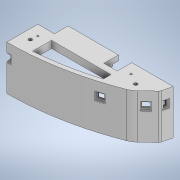
# Autodesk Inventor part: bumper_base_final _원본수정
Saved by Autodesk Inventor 2020 (Build 240168000, 168)
## iProperties
Created: 2022-06-30
Part Number: bumper_base_final _원본수정
Material: 일반
Document SubType Name: Modeling
Designer: samsung
Density: 1 g/cm^3
Appearance: 기본값
Author: samsung
Autodesk Inventor part; units mm, degrees
sketch "스케치1" plane through (0, 0, 0) normal (0, 1, 0) x (-1, 0, 0)
  line L0 (-417.5, 136.0278) -> (167.5, 136.0278)
  line L1 (143.8982, 68.5278) -> (-85, 68.5278)
  line L2 (-165, 68.5278) -> (-381.3624, 68.5278)
  line L3 (-125, -531.4722) -> (-125, 1435.9267)
  circle A0 centre (-125, -531.4722) radius 1967.3989
  line L4 (-125, 111.6599) -> (186.953, 1411.0375)
  line L5 (-417.5444, 28.5399) -> (-411.5443, 53.4914)
  arc A1 (1441.9544, 38.2515) -> (-1691.7763, 38.7413) centre (-125, -531.4722) ccw
  line L6 (-371.3038, 78.1512) -> (-261.7019, 111.6599)
  line L7 (-261.7019, 111.6599) -> (11.7019, 111.6599)
  line L8 (-316.5029, 94.9056) -> (-320.1581, 106.8613)
  line L9 (-407.5098, 28.5399) -> (-405.1717, 38.2627)
  line L10 (-405.1717, 38.2627) -> (-402.8337, 47.9856)
  line L11 (-402.8337, 47.9856) -> (-371.3038, 78.1512)
  line L12 (-125, -531.4722) -> (-261.7019, 111.6599)
  line L13 (-125, -531.4722) -> (11.7019, 111.6599)
  line L14 (-417.5444, 28.5399) -> (-407.5098, 28.5399)
  line L15 (-125, -531.4722) -> (-371.3038, 78.1512)
  line L16 (-125, -531.4722) -> (121.3038, 78.1512)
  line L17 (11.7019, 111.6599) -> (121.3038, 78.1512)
  line L18 (167.4556, 28.5399) -> (156.6099, 73.7155)
  line L19 (157.5156, 28.5399) -> (148.4052, 66.4876)
  line L20 (121.3038, 78.1512) -> (152.8486, 47.9794)
  line L21 (155.1841, 38.2515) -> (1758.102, 38.2515)
  line L22 (155.1841, 38.2515) -> (164.5823, 40.5079)
  line L23 (157.5156, 28.5399) -> (167.4556, 28.5399)
  line L24 (155.1841, 38.2515) -> (1422.1711, 683.8137)
  line L25 (66.5029, 94.9056) -> (70.1581, 106.8613)
  line L26 (66.5029, 94.9056) -> (738.7616, 1236.1743)
  line L27 (66.5029, 94.9056) -> (147.3646, 1416.9826)
  line L28 (137.0762, 63.0653) -> (150.1137, 76.6961)
  line L29 (137.0762, 63.0653) -> (801.7772, 1203.965)
  line L30 (137.0762, 63.0653) -> (1307.7755, 816.7906)
  line L31 (-125, -531.4722) -> (148.4052, 66.4876)
  line L32 (-259.0118, 93.6599) -> (9.0118, 93.6599)
  line L33 (111.9521, 62.1879) -> (136.5817, 38.6304)
  line L34 (9.0118, 93.6599) -> (111.9521, 62.1879)
  line L35 (-361.9509, 62.1883) -> (-386.641, 38.5664)
  line L36 (-387.0049, 38.256) -> (-387.0101, 38.2515)
  line L37 (-388.9967, 28.5399) -> (-386.569, 38.6353)
  line L38 (-361.9509, 62.1883) -> (-259.0118, 93.6599)
  line L39 (-407.5098, 28.5399) -> (-388.9967, 28.5399)
  line L40 (136.5817, 38.6304) -> (139.0042, 28.5399)
  line L41 (157.5156, 28.5399) -> (139.0042, 28.5399)
  line L42 (-125, 111.6599) -> (-155, 111.6599)
  line L43 (-155, 93.6599) -> (-125, 93.6599)
  line L44 (-125, 93.6599) -> (-125, 111.6599)
  line L45 (-376.8352, 86.6988) -> (-411.5443, 53.4914)
  arc A2 (156.6099, 73.7155) -> (-376.8352, 86.6988) centre (-125, -531.4722) ccw
  arc A3 (148.4052, 66.4876) -> (-371.3038, 78.1512) centre (-125, -531.4722) ccw
  arc A4 (-398.3819, 66.4982) -> (-398.3844, 66.4971) centre (-125, -531.4722) ccw
  line L46 (-407.5098, 28.5399) -> (-402.8337, 47.9856)
  line L47 (-398.3829, 66.4939) -> (-398.3801, 66.5058)
  line L48 (-398.3844, 66.4971) -> (-398.2523, 66.2083)
  line L49 (-393.8505, 56.5801) -> (-125, -531.4722)
  line L50 (-125, 111.6599) -> (-135, 111.6599)
  line L51 (-135, 111.6599) -> (-135, 103.6599)
  line L52 (-135, 103.6599) -> (-125, 103.6599)
  line L53 (-316.5029, 94.9056) -> (-326.0659, 91.9818)
  line L54 (-326.0659, 91.9818) -> (-323.727, 84.3314)
  line L55 (-323.727, 84.3314) -> (-304.6009, 90.1788)
  line L56 (-304.6009, 90.1788) -> (-306.9398, 97.8293)
  line L57 (-402.8337, 47.9856) -> (-395.0554, 46.1151)
  line L58 (-395.0554, 46.1151) -> (-398.5625, 31.5309)
  line L59 (-398.5625, 31.5309) -> (-406.3408, 33.4013)
  line L60 (-387.0687, 63.0684) -> (-394.2944, 56.1554)
  line L61 (-394.2944, 56.1554) -> (-388.764, 50.3749)
  line L62 (-388.764, 50.3749) -> (-374.3127, 64.2009)
  line L63 (-374.3127, 64.2009) -> (-379.8431, 69.9814)
  line L64 (-165, 0) -> (-165, 124.81)
  line L65 (-341.215, 68.5278) -> (-341.215, 89.4604)
  line L66 (-388.9967, 28.5399) -> (-125, 28.5399)
  line L67 (-125, 0) -> (-165, 0)
  line L68 (-175, 28.5399) -> (-175, 124.1239)
  line L69 (-165, 0) -> (-135, 0)
  line L70 (-135, 0) -> (-135, 61.5)
  line L71 (-135, 61.5) -> (-165, 61.5)
  line L72 (-165, 61.5) -> (-165, 0)
  line L73 (-165, 61.5) -> (-175, 61.5)
  line L74 (-135, 61.5) -> (-125, 61.5)
  line L75 (-175, 78.5399) -> (-370.0325, 78.5399)
  line L76 (-318, 28.5399) -> (-318, 97.0636)
  line L77 (-286, 28.5399) -> (-286, 89.4604)
  line L78 (-318, 28.5399) -> (-318, 94.4478)
  line L79 (-286, 28.5399) -> (-318, 28.5399)
  line L80 (-318, 28.5399) -> (-318, 63.5399)
  line L81 (-318, 63.5399) -> (-286, 63.5399)
  line L82 (-286, 63.5399) -> (-286, 28.5399)
  point P0 (0, 0)
  point P1 (0, 0)
  point P2 (143.8982, 61.5)
  point P3 (-393.8982, 61.5)
  point P4 (-417.5, 21.5)
  point P5 (-165, 0)
  point P6 (-85, 0)
  point P7 (-85, 12.4229)
  point P8 (167.5, 12.4229)
  point P9 (-393.8982, -388.5)
  point P10 (-165, -388.5)
  point P11 (167.5, -327)
  point P12 (-417.5, -327)
  point P13 (-85, -388.5)
  point P14 (143.8982, -388.5)
  point P15 (162, 21.5)
  point P16 (162, 12.4229)
  point P17 (167.5, 21.5)
  point P18 (-125, 0)
  point P19 (-125, 136.0278)
  point P20 (-125, 136.0278)
  point P21 (-125, 93.6599)
  point P22 (-125, 126.0278)
  point P23 (-317.2344, 97.2982)
  point P24 (-378.4524, 68.5278)
  point P25 (-393.0723, 54.878)
  point P26 (-175, 68.5278)
  point P27 (-341.215, 78.5399)
  point P28 (-351.2596, 28.5399)
  point P29 (-318, 68.5278)
  point P30 (-318, 94.4478)
  point P31 (-165, 28.5399)
  point P32 (-308.467, 78.5399)
  point P33 (-318, 75.6254)
  point P34 (-318, 78.5399)
  point P35 (-286, 68.5278)
  dimension "d15" = 585
  dimension "d31" = 13.5
  dimension "d56" = 12
  dimension "d57" = 12
  dimension "d60" = 10
  dimension "d65" = 13.5
  dimension "d66" = 13.5
  dimension "d68" = 13.5
  dimension "d69" = 13.5
  dimension "d70" = 13.5
  dimension "d71" = 13.5
  dimension "d72" = 10
  dimension "d81" = 18
  dimension "d83" = 18
  dimension "d84" = 18
  dimension "d85" = 18
  dimension "d86" = 18
  dimension "d159" = 10
  dimension "d164" = 10
  dimension "d165" = 8
  dimension "d166" = 10
  dimension "d167" = 8
  dimension "d168" = 20
  dimension "d169" = 8
  dimension "d170" = 15
  dimension "d171" = 10
  dimension "d172" = 8
  dimension "d173" = 20
  dimension "d191" = 30
  dimension "d192" = 61.5
  dimension "d194" = 50
  dimension "d256" = 143
  dimension "d264" = 121
  dimension "d265" = 32
  dimension "d266" = 35
  constraints: 166 end point, 33 point on line, 22 perpendicular, 14 parallel, 11 horizontal, 10 point on circle, 7 midpoint, 3 centre point, 2 vertical, 1 coincident, 1 tangent, 23 other
  measures "d15" distance of L18.start L5.start
  measures "d31" angle of L4 L3
  measures "d56" angle of L3 L12
  measures "d57" angle of L13 L3
  measures "d60" angle of L15 L12
  measures "d65" angle of L22 L21
  measures "d66" angle of L24 L22
  measures "d68" angle of L26 L25
  measures "d69" angle of L25 L27
  measures "d70" angle of L29 L28
  measures "d71" angle of L30 L28
  measures "d72" angle of L16 L13
  measures "d81" distance between parallel lines of L7 L32
  measures "d83" distance between parallel lines of L20 L33
  measures "d84" distance between parallel lines of L11 L35
  measures "d85" distance between parallel lines of L9 L37
  measures "d86" distance between parallel lines of L19 L40
  measures "d159" distance between parallel lines of L11 L45
  measures "d164" distance of L4.start L50.end
  measures "d165" distance of L50.end L51.end
  measures "d166" distance of L8.start L53.end
  measures "d167" distance of L53.end L54.end
  measures "d168" distance of L54.end L55.end
  measures "d169" distance of L10.end L57.end
  measures "d170" distance of L57.end L58.end
  measures "d171" distance of L60.start L60.end
  measures "d172" distance of L60.end L61.end
  measures "d173" distance of L61.end L62.end
  measures "d191" distance of L71.end L70.end
  measures "d192" distance of L70.end L69.end
  measures "d194" distance between parallel lines of L66 L75
  measures "d256" distance between parallel lines of L68 L76
  measures "d264" distance between parallel lines of L77 L64
  measures "d265" distance between parallel lines of L78 L77
  measures "d266" distance of L79.end L80.end
extrude "돌출11" add sketch "스케치1" against normal blind 90 contours L3 A3 L8 A2 | L8 A3 L11 L10 L9 L14 L5 L45 A2
ref_plane "작업 평면1" through (125, 0, 103.6599) normal (0, 0, 1) x (1, 0, 0)
sketch "스케치14" plane through (125, 0, 103.6599) normal (0, 0, 1) x (1, 0, 0)
  line L0 (0, 0) -> (10, 0) projected
  line L1 (10, -30) -> (0, -30) projected
  line L2 (7.5, -7.5) -> (-7.5, -7.5)
  line L3 (-7.5, -7.5) -> (-7.5, -22.5)
  line L4 (-7.5, -22.5) -> (7.5, -22.5)
  line L5 (7.5, -22.5) -> (7.5, -7.5)
  line L6 (7.5, -7.5) -> (-7.5, -22.5) construction
  line L7 (-7.5, -7.5) -> (7.5, -22.5) construction
  line L8 (0, -7.5) -> (0, -22.5)
  point P0 (0, -15)
  dimension "d236" = 15
  dimension "d237" = 15
  constraints: 14 end point, 4 midpoint, 2 parallel, 1 horizontal, 1 perpendicular
  measures "d236" distance of L4.end L3.end
  measures "d237" distance of L3.end L2.end
extrude "돌출13" cut sketch "스케치14" along normal blind 50 contours L5 L4 L8 L2
ref_plane "작업 평면2" through (304.6009, -30, 90.1788) normal (0.2923717, 0, 0.9563048) x (0.9563048, 0, -0.2923717)
sketch "스케치15" plane through (304.6009, -30, 90.1788) normal (0.2923717, 0, 0.9563048) x (0.9563048, 0, -0.2923717)
  line L0 (0, 30) -> (20, 30)
  line L1 (0, 30) -> (0, 0)
  line L2 (20, 0) -> (0, 0)
  line L3 (20, 30) -> (20, 0)
  line L4 (2.5, 22.5) -> (17.5, 22.5)
  line L5 (17.5, 22.5) -> (17.5, 7.5)
  line L6 (17.5, 7.5) -> (2.5, 7.5)
  line L7 (2.5, 7.5) -> (2.5, 22.5)
  line L8 (2.5, 22.5) -> (17.5, 7.5) construction
  line L9 (17.5, 22.5) -> (2.5, 7.5) construction
  point P0 (-264.9255, 30)
  point P1 (10, 15)
  dimension "d234" = 15
  dimension "d235" = 15
  constraints: 20 end point, 2 midpoint, 2 parallel, 1 horizontal, 1 perpendicular
  measures "d234" distance of L5.end L6.end
  measures "d235" distance of L4.end L5.end
extrude "돌출14" cut sketch "스케치15" along normal blind 50 contours L4 L5 L6 L7
ref_plane "작업 평면3" through (374.3127, -30, 64.2009) normal (0.6913026, 0, 0.7225653) x (0.7225653, 0, -0.6913026)
sketch "스케치16" plane through (374.3127, -30, 64.2009) normal (0.6913026, 0, 0.7225653) x (0.7225653, 0, -0.6913026)
  line L0 (0, 30) -> (20, 30)
  line L1 (0, 30) -> (0, 0)
  line L2 (20, 0) -> (0, 0)
  line L3 (20, 30) -> (20, 0)
  line L4 (2.5, 22.5) -> (17.5, 22.5)
  line L5 (17.5, 22.5) -> (17.5, 7.5)
  line L6 (17.5, 7.5) -> (2.5, 7.5)
  line L7 (2.5, 7.5) -> (2.5, 22.5)
  line L8 (2.5, 22.5) -> (17.5, 7.5) construction
  line L9 (17.5, 22.5) -> (2.5, 7.5) construction
  point P0 (-226.0831, 30)
  point P1 (10, 15)
  dimension "d232" = 15
  dimension "d233" = 15
  constraints: 20 end point, 2 midpoint, 2 parallel, 1 horizontal, 1 perpendicular
  measures "d232" distance of L5.end L6.end
  measures "d233" distance of L4.end L5.end
extrude "돌출15" cut sketch "스케치16" along normal blind 50 contours L4 L5 L6 L7
ref_plane "작업 평면4" through (395.0554, -30, 46.1151) normal (0.972283, 0, 0.233807) x (0.233807, 0, -0.972283)
sketch "스케치17" plane through (395.0554, -30, 46.1151) normal (0.972283, 0, 0.233807) x (0.233807, 0, -0.972283)
  line L0 (0, 30) -> (15, 30)
  line L1 (0, 30) -> (0, 0)
  line L2 (15, 0) -> (0, 0)
  line L3 (15, 30) -> (15, 0)
  line L4 (11.5, 22.5) -> (3.5, 22.5)
  line L5 (3.5, 22.5) -> (3.5, 7.5)
  line L6 (3.5, 7.5) -> (11.5, 7.5)
  line L7 (11.5, 7.5) -> (11.5, 22.5)
  line L8 (11.5, 22.5) -> (3.5, 7.5) construction
  line L9 (3.5, 22.5) -> (11.5, 7.5) construction
  point P0 (7.5, 15)
  point P1 (7.5, 15)
  point P2 (15, 15)
  dimension "d230" = 8
  dimension "d231" = 15
  constraints: 20 end point, 4 midpoint, 2 parallel, 1 horizontal, 1 horizontal alignment, 1 perpendicular, 4 other
  measures "d230" distance of L6.end L5.end
  measures "d231" distance of L5.end L4.end
extrude "돌출16" cut sketch "스케치17" along normal blind 50 contours L7 L6 L5 L4
extrude "돌출17" add sketch "스케치1" along normal blind 17 contours L3 A3 L8 A2 | L3 L7 L64 A3 | L8 A3 L11 L10 L9 L14 L5 L45 A2 | L3 L52 L51 L7 | L64 L7 L68 A3 | L3 L32 L64 L7 L51 L52 | L64 L32 L68 L7 | L76 L6 L65 A3 | L3 L74 L71 L64 L32 | L64 L2 L68 L32 | L76 L55 L54 L6 | L65 L6 A3 | L64 L73 L68 L2 | L54 L55 L76 L75 L65 L6 | L75 L68 L2 L12 | L12 L2 L77 L75 | L15 L2 L63 L11 | L6 L75 L65 L2 L15 | L65 L75 L6 | L68 L66 L12 L2 | L64 L66 L68 L73 | L76 L38 L65 L75 | L75 L38 L76 | L12 L66 L77 L2 | L77 L2 L76 L38 L75 | L63 L2 L11 | L15 L35 L49 L61 L62 L63 L2 | L2 L38 L35 L15 | L9 L59 L58 L57 L11 L61 L49 L35 L37 L39 | L66 L49 L35 L15 | L15 L35 L38 L2 L76 L66 | L66 L37 L35 L49 | L76 L2 L38 | L77 L81 L76 L2 | L2 L63 L62 L61 L49 L11 | L9 L10 L57 L58 L59 | L61 L11 L49
sketch "스케치18" plane through (0, 17, 0) normal (0, 1, 0) x (1, 0, 0)
  line L0 (407.5098, -28.5399) -> (402.8337, -47.9856) projected
  line L1 (402.8337, -47.9856) -> (371.3038, -78.1512) projected
  arc A0 (125, -126.0278) -> (371.3038, -78.1512) centre (125, 531.4722) ccw projected
  line L2 (417.5444, -28.5399) -> (318, -28.5399) projected
  circle A1 centre (367.5098, -68.5399) radius 3.6
  line L3 (369.5883, -64.9399) -> (371.6667, -68.5399)
  line L4 (371.6667, -68.5399) -> (369.5883, -72.1399)
  line L5 (369.5883, -72.1399) -> (365.4313, -72.1399)
  line L6 (365.4313, -72.1399) -> (363.3529, -68.5399)
  line L7 (363.3529, -68.5399) -> (365.4313, -64.9399)
  line L8 (365.4313, -64.9399) -> (369.5883, -64.9399)
  line L9 (261.7019, -111.6599) -> (-11.7019, -111.6599) projected
  line L10 (259.0118, -93.6599) -> (-9.0118, -93.6599) projected
  line L11 (125, 531.4722) -> (125, -126.0278) projected
  line L12 (125, 202.7222) -> (125, -111.6599)
  circle A2 centre (148, -102.6599) radius 3.6
  line L13 (150.0785, -99.0599) -> (152.1569, -102.6599)
  line L14 (152.1569, -102.6599) -> (150.0785, -106.2599)
  line L15 (150.0785, -106.2599) -> (145.9215, -106.2599)
  line L16 (145.9215, -106.2599) -> (143.8431, -102.6599)
  line L17 (143.8431, -102.6599) -> (145.9215, -99.0599)
  line L18 (145.9215, -99.0599) -> (150.0785, -99.0599)
  point P0 (0, 0)
  point P1 (341.215, -89.4604)
  point P2 (165, -28.5399)
  point P3 (367.5098, -64.9399)
  point P4 (125, -61.5)
  point P5 (148, -99.0599)
  point P6 (175, -124.1239)
  point P7 (351.2596, -28.5399)
  dimension "d197" = 7.2
  dimension "d229" = 7.2
  dimension "d195" = 40
  dimension "d196" = 40
  dimension "d224" = 9
  dimension "d225" = 23
  constraints: 26 end point, 5 coincident, 4 midpoint, 2 vertical alignment, 1 point on line, 30 other
  measures "d195" horizontal distance of point (367.51, -68.54) L0.start
  measures "d196" horizontal distance of L0.start point (367.51, -68.54)
  measures "d224" distance from line of point (148, -102.66) L9
  measures "d225" distance from line of point (148, -102.66) L11
extrude "돌출18" cut sketch "스케치18" against normal blind 10 contours A1 | A1 L3 L4 | A1 L8 L3 | L4 L5 A1 | A1 L7 L8 | L5 L6 A1 | A1 L6 L7 | A2 | A2 L13 L14 | A2 L18 L13 | L14 L15 A2 | A2 L17 L18 | L15 L16 A2 | A2 L16 L17
sketch "스케치19" plane through (0, 7, 0) normal (0, 1, 0) x (1, 0, 0)
  line L0 (363.3529, -68.5399) -> (365.4313, -64.9399) projected
  line L1 (365.4313, -72.1399) -> (363.3529, -68.5399) projected
  line L2 (369.5883, -72.1399) -> (365.4313, -72.1399) projected
  line L3 (371.6667, -68.5399) -> (369.5883, -72.1399) projected
  line L4 (369.5883, -64.9399) -> (371.6667, -68.5399) projected
  line L5 (365.4313, -64.9399) -> (369.5883, -64.9399) projected
  line L6 (125, -61.5) -> (125, -126.0278) projected
  line L7 (261.7019, -111.6599) -> (-11.7019, -111.6599) projected
  line L8 (259.0118, -93.6599) -> (-9.0118, -93.6599) projected
  line L9 (152.1569, -102.6599) -> (150.0785, -106.2599) projected
  line L10 (150.0785, -99.0599) -> (152.1569, -102.6599) projected
  line L11 (145.9215, -99.0599) -> (150.0785, -99.0599) projected
  line L12 (143.8431, -102.6599) -> (145.9215, -99.0599) projected
  line L13 (145.9215, -106.2599) -> (143.8431, -102.6599) projected
  line L14 (150.0785, -106.2599) -> (145.9215, -106.2599) projected
  point P0 (0, 0)
  point P1 (367.5098, -68.5399)
  point P2 (148, -102.6599)
  point P3 (125, 531.4722)
  point P4 (125, 0)
  point P5 (125, -28.5399)
  dimension "d227" = 23
  dimension "d228" = 9
  measures "d227" distance from line of L6 point (148, -102.66)
  measures "d228" distance from line of L8 point (148, -102.66)
hole "구멍3" at (367.5098, 7, 68.5399) at (148, 7, 102.6599) direction (0, -1, 0) diameter 4.2 end through all
sketch "스케치20" plane through (0, 0, 0) normal (0, -1, 0) x (1, 0, 0)
  circle A0 centre (367.5098, 68.5399) radius 2.1 projected
  arc A1 (175, 124.1239) -> (125, 126.0278) centre (125, -531.4722) ccw projected
  line L0 (125, 61.5) -> (125, 126.0278) projected
  line L1 (407.5098, 28.5399) -> (402.8337, 47.9856) projected
  line L2 (402.8337, 47.9856) -> (371.3038, 78.1512) projected
  circle A2 centre (150, 86.5) radius 3.6
  circle A3 centre (341.215, 53.5399) radius 3.6
  line L3 (152.0785, 90.1) -> (154.1569, 86.5)
  line L4 (154.1569, 86.5) -> (152.0785, 82.9)
  line L5 (152.0785, 82.9) -> (147.9215, 82.9)
  line L6 (147.9215, 82.9) -> (145.8431, 86.5)
  line L7 (145.8431, 86.5) -> (147.9215, 90.1)
  line L8 (147.9215, 90.1) -> (152.0785, 90.1)
  line L9 (343.2935, 57.1399) -> (345.372, 53.5399)
  line L10 (345.372, 53.5399) -> (343.2935, 49.9399)
  line L11 (343.2935, 49.9399) -> (339.1366, 49.9399)
  line L12 (339.1366, 49.9399) -> (337.0581, 53.5399)
  line L13 (337.0581, 53.5399) -> (339.1366, 57.1399)
  line L14 (339.1366, 57.1399) -> (343.2935, 57.1399)
  line L15 (175, 124.1239) -> (175, 78.5399) projected
  arc A4 (371.3038, 78.1512) -> (318, 97.0636) centre (125, -531.4722) ccw projected
  line L16 (165, 61.5) -> (125, 61.5) projected
  circle A5 centre (148, 102.6599) radius 2.1 projected
  line L17 (165, 28.5399) -> (165, 61.5) projected
  line L18 (286, 28.5399) -> (165, 28.5399) projected
  line L19 (175, 78.5399) -> (318, 78.5399) projected
  line L20 (286, 63.5399) -> (286, 28.5399) projected
  line L21 (407.5098, 28.5399) -> (318, 28.5399) projected
  line L22 (318, 63.5399) -> (286, 63.5399) projected
  line L23 (318, 28.5399) -> (318, 63.5399) projected
  line L24 (318, 78.5399) -> (318, 97.0636) projected
  point P0 (0, 0)
  point P1 (341.215, 84.0002)
  point P2 (150, 90.1)
  point P3 (341.215, 57.1399)
  dimension "d212" = 7.2
  dimension "d213" = 7.2
  dimension "d259" = 25
  dimension "d263" = 25
  constraints: 24 end point, 5 coincident, 3 vertical alignment, 2 midpoint, 30 other
  measures "d259" distance from line of L0 point (150, 86.5)
  measures "d263" distance from line of L16 point (150, 86.5)
extrude "돌출19" cut sketch "스케치20" against normal blind 10 contours A2 | A2 L3 L4 | A2 L8 L3 | L4 L5 A2 | A2 L7 L8 | L5 L6 A2 | A2 L6 L7 | A3 | A3 L9 L10 | A3 L14 L9 | L10 L11 A3 | A3 L13 L14 | L11 L12 A3 | A3 L12 L13
sketch "스케치21" plane through (0, 10, 0) normal (0, -1, 0) x (1, 0, 0)
  line L0 (147.9215, 90.1) -> (152.0785, 90.1) projected
  line L1 (145.8431, 86.5) -> (147.9215, 90.1) projected
  line L2 (147.9215, 82.9) -> (145.8431, 86.5) projected
  line L3 (152.0785, 82.9) -> (147.9215, 82.9) projected
  line L4 (154.1569, 86.5) -> (152.0785, 82.9) projected
  line L5 (152.0785, 90.1) -> (154.1569, 86.5) projected
  line L6 (339.1366, 49.9399) -> (337.0581, 53.5399) projected
  line L7 (343.2935, 49.9399) -> (339.1366, 49.9399) projected
  line L8 (345.372, 53.5399) -> (343.2935, 49.9399) projected
  line L9 (343.2935, 57.1399) -> (345.372, 53.5399) projected
  line L10 (339.1366, 57.1399) -> (343.2935, 57.1399) projected
  line L11 (337.0581, 53.5399) -> (339.1366, 57.1399) projected
  circle A0 centre (148, 102.6599) radius 2.1 projected
  arc A1 (175, 124.1239) -> (125, 126.0278) centre (125, -531.4722) ccw projected
  line L12 (125, 61.5) -> (125, 126.0278) projected
  line L13 (165, 61.5) -> (125, 61.5) projected
  line L14 (175, 124.1239) -> (175, 78.5399) projected
  line L15 (165, 28.5399) -> (165, 61.5) projected
  line L16 (286, 28.5399) -> (165, 28.5399) projected
  line L17 (407.5098, 28.5399) -> (402.8337, 47.9856) projected
  line L18 (402.8337, 47.9856) -> (371.3038, 78.1512) projected
  arc A2 (371.3038, 78.1512) -> (318, 97.0636) centre (125, -531.4722) ccw projected
  line L19 (175, 78.5399) -> (318, 78.5399) projected
  line L20 (286, 63.5399) -> (286, 28.5399) projected
  line L21 (407.5098, 28.5399) -> (318, 28.5399) projected
  line L22 (318, 63.5399) -> (286, 63.5399) projected
  line L23 (318, 28.5399) -> (318, 63.5399) projected
  line L24 (318, 78.5399) -> (318, 97.0636) projected
  point P0 (0, 0)
  point P1 (150, 86.5)
  point P2 (341.215, 53.5399)
  dimension "d260" = 25
  dimension "d261" = 25
  measures "d260" distance from line of L12 point (150, 86.5)
  measures "d261" distance from line of L13 point (150, 86.5)
hole "구멍4" at (150, 10, 86.5) at (341.215, 10, 53.5399) direction (0, 1, 0) diameter 4.2 end through all
sketch "스케치22" plane through (411.5443, -90, 53.4914) normal (0.972283, 0, 0.233807) x (0.233807, 0, -0.972283)
  line L0 (6.8166, 82.5) -> (14.8166, 82.5) projected
  line L1 (6.8166, 67.5) -> (6.8166, 82.5) projected
  line L2 (14.8166, 67.5) -> (6.8166, 67.5) projected
  line L3 (14.8166, 82.5) -> (14.8166, 67.5) projected
  line L4 (3.3166, 85) -> (18.3166, 85)
  line L5 (18.3166, 85) -> (18.3166, 65)
  line L6 (18.3166, 65) -> (3.3166, 65)
  line L7 (3.3166, 65) -> (3.3166, 85)
  line L8 (3.3166, 85) -> (18.3166, 65) construction
  line L9 (18.3166, 85) -> (3.3166, 65) construction
  point P0 (10.8166, 75)
  dimension "d238" = 15
  dimension "d239" = 20
  constraints: 12 end point, 2 midpoint, 2 parallel, 1 horizontal, 1 perpendicular
  measures "d238" distance of L5.end L6.end
  measures "d239" distance of L4.end L5.end
extrude "돌출20" cut sketch "스케치22" against normal blind 2 contours L0 L3 L2 L1 | L4 L5 L6 L7
sketch "스케치23" plane through (376.8352, -90, 86.6988) normal (0.6913026, 0, 0.7225653) x (0.7225653, 0, -0.6913026)
  line L0 (16.2301, 67.5) -> (16.2301, 82.5) projected
  line L1 (16.2301, 82.5) -> (31.2301, 82.5) projected
  line L2 (31.2301, 82.5) -> (31.2301, 67.5) projected
  line L3 (31.2301, 67.5) -> (16.2301, 67.5) projected
  line L4 (13.7301, 85) -> (33.7301, 85)
  line L5 (33.7301, 85) -> (33.7301, 65)
  line L6 (33.7301, 65) -> (13.7301, 65)
  line L7 (13.7301, 65) -> (13.7301, 85)
  line L8 (13.7301, 85) -> (33.7301, 65) construction
  line L9 (33.7301, 85) -> (13.7301, 65) construction
  point P0 (23.7301, 75)
  dimension "d242" = 20
  dimension "d243" = 20
  constraints: 12 end point, 2 midpoint, 2 parallel, 1 horizontal, 1 perpendicular
  measures "d242" distance of L5.end L6.end
  measures "d243" distance of L4.end L5.end
extrude "돌출21" cut sketch "스케치23" against normal blind 2 contours L0 L1 L2 L3 | L4 L5 L6 L7
ref_plane "작업 평면5" through (312.9735, -7.5, 109.0138) normal (-0.2923717, 0, -0.9563048) x (0.9563048, 0, -0.2923717)
sketch "스케치24" plane through (312.9735, -7.5, 109.0138) normal (-0.2923717, 0, -0.9563048) x (0.9563048, 0, -0.2923717)
  line L0 (0, 15) -> (0, 0) projected
  line L1 (0, 0) -> (15, 0) projected
  line L2 (15, 0) -> (15, 15) projected
  line L3 (15, 15) -> (0, 15) projected
  line L4 (-2.5, -2.5) -> (17.5, -2.5)
  line L5 (17.5, -2.5) -> (17.5, 17.5)
  line L6 (17.5, 17.5) -> (-2.5, 17.5)
  line L7 (-2.5, 17.5) -> (-2.5, -2.5)
  line L8 (-2.5, -2.5) -> (17.5, 17.5) construction
  line L9 (17.5, -2.5) -> (-2.5, 17.5) construction
  point P0 (-267.4255, -7.5)
  point P1 (7.5, 7.5)
  dimension "d246" = 20
  dimension "d247" = 20
  constraints: 12 end point, 2 midpoint, 2 parallel, 1 horizontal, 1 perpendicular
  measures "d246" distance of L6.end L5.end
  measures "d247" distance of L5.end L4.end
extrude "돌출22" cut sketch "스케치24" along normal mid plane 4 contours L3 L2 L1 L0 | L7 L6 L5 L4
ref_plane "작업 평면6" through (132.5, -7.5, 135.9857) normal (0.0056181, 0, 0.9999842) x (-0.9999842, 0, 0.0056181)
sketch "스케치25" plane through (132.5, -7.5, 135.9857) normal (0.0056181, 0, 0.9999842) x (-0.9999842, 0, 0.0056181)
  line L0 (0, 0) -> (7.5001, 0) projected
  line L1 (0, 0) -> (0, 15) projected
  line L2 (7.5001, 15) -> (0, 15) projected
  line L3 (17.5001, -2.5) -> (-2.4999, -2.5)
  line L4 (-2.4999, -2.5) -> (-2.4999, 17.5)
  line L5 (-2.4999, 17.5) -> (17.5001, 17.5)
  line L6 (17.5001, 17.5) -> (17.5001, -2.5)
  line L7 (17.5001, -2.5) -> (-2.4999, 17.5) construction
  line L8 (-2.4999, -2.5) -> (17.5001, 17.5) construction
  line L9 (7.5001, 0) -> (7.5001, -24.5) projected
  line L10 (7.5001, -2.5) -> (7.5001, 17.5)
  point P0 (7.5001, 7.5)
  point P1 (7.5001, 0)
  dimension "d250" = 20
  dimension "d251" = 20
  constraints: 14 end point, 4 midpoint, 2 parallel, 1 horizontal, 1 perpendicular, 1 point on line
  measures "d250" distance of L4.end L5.end
  measures "d251" distance of L3.end L4.end
extrude "돌출23" cut sketch "스케치25" along normal mid plane 4 contours L1 L2 L10 L0 | L0 L9 L3 L4 L5 L10 L2 L1
fillet "모깎기1" radius 50 1 edges at (376.8352, -36.5, 86.6988)
fillet "모깎기2" radius 10 1 edges at (411.5443, -36.5, 53.4914)
sketch "스케치26" plane through (0, 0, 0) normal (0, -1, 0) x (1, 0, 0)
  line L0 (343.2935, 57.1399) -> (345.372, 53.5399) projected
  line L1 (345.372, 53.5399) -> (343.2935, 49.9399) projected
  line L2 (343.2935, 49.9399) -> (339.1366, 49.9399) projected
  line L3 (339.1366, 49.9399) -> (337.0581, 53.5399) projected
  line L4 (337.0581, 53.5399) -> (339.1366, 57.1399) projected
  line L5 (339.1366, 57.1399) -> (343.2935, 57.1399) projected
  line L6 (154.1569, 86.5) -> (152.0785, 82.9) projected
  line L7 (152.0785, 82.9) -> (147.9215, 82.9) projected
  line L8 (147.9215, 82.9) -> (145.8431, 86.5) projected
  line L9 (145.8431, 86.5) -> (147.9215, 90.1) projected
  line L10 (147.9215, 90.1) -> (152.0785, 90.1) projected
  line L11 (152.0785, 90.1) -> (154.1569, 86.5) projected
  circle A0 centre (367.5098, 68.5399) radius 2.1 projected
  circle A1 centre (148, 102.6599) radius 2.1 projected
  arc A2 (175, 124.1239) -> (125, 126.0278) centre (125, -531.4722) ccw projected
  line L12 (125, 61.5) -> (125, 126.0278) projected
  line L13 (165, 61.5) -> (125, 61.5) projected
  line L14 (165, 28.5399) -> (165, 61.5) projected
  line L15 (286, 28.5399) -> (165, 28.5399) projected
  line L16 (286, 63.5399) -> (286, 28.5399) projected
  line L17 (318, 63.5399) -> (286, 63.5399) projected
  line L18 (407.5098, 28.5399) -> (318, 28.5399) projected
  line L19 (407.5098, 28.5399) -> (402.8337, 47.9856) projected
  line L20 (402.8337, 47.9856) -> (371.3038, 78.1512) projected
  arc A3 (371.3038, 78.1512) -> (318, 97.0636) centre (125, -531.4722) ccw projected
  line L21 (175, 78.5399) -> (318, 78.5399) projected
  line L22 (175, 124.1239) -> (175, 78.5399) projected
  line L23 (318, 28.5399) -> (318, 63.5399) projected
  line L24 (318, 78.5399) -> (318, 97.0636) projected
  line L25 (165, 28.5399) -> (165, 61.5) projected
  line L26 (286, 63.5399) -> (286, 28.5399) projected
  line L27 (165, 28.5399) -> (286, 28.5399)
  line L28 (286, 28.5399) -> (286, 42.5399)
  line L29 (286, 42.5399) -> (165, 42.5399)
  line L30 (165, 42.5399) -> (165, 28.5399)
  point P0 (0, 0)
  dimension "d267" = 14
  constraints: 8 end point, 2 parallel, 1 horizontal, 1 perpendicular, 1 point on line
  measures "d267" distance of L28.end L27.end
extrude "돌출24" cut sketch "스케치26" against normal blind 4.7 contours L29 L16 L15 L14
equation "\"d57\" = d56"
equation "\"d72\" = d60"
equation "\"d61\" = d60"
